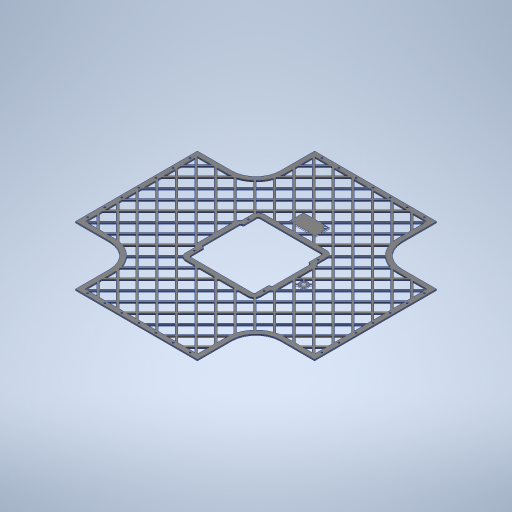
# Autodesk Inventor part: Swerve-Electronic-Pannel
Saved by Autodesk Inventor 2024.2 (Build 282272000, 272)
## iProperties
Created: 2024-01-04
Part Number: Swerve-Electronic-Pannel
Material: Aluminum 6061
Document SubType Name: Modeling
Designer: rohan
Density: 2.7 g/cm^3
Appearance: Aluminum - Flat
Author: rohan
Autodesk Inventor part; units mm, degrees
(part 1 of 6)
ref_plane "YZ Plane" through (0, 0, 0) normal (1, 0, 0) x (0, 1, 0)
ref_plane "XZ Plane" through (0, 0, 0) normal (0, 1, 0) x (-1, 0, 0)
ref_plane "XY Plane" through (0, 0, 0) normal (0, 0, 1) x (1, 0, 0)
sketch "Sketch6" plane through (0, 0, 0) normal (0, 1, 0) x (-1, 0, 0)
  line L0 (311.15, 311.15) -> (-311.15, 311.15)
  line L1 (-311.15, 311.15) -> (-311.15, -311.15)
  line L2 (-311.15, -311.15) -> (311.15, -311.15)
  line L3 (311.15, -311.15) -> (311.15, 311.15)
  line L4 (311.15, 311.15) -> (-311.15, -311.15) construction
  line L5 (-311.15, 311.15) -> (311.15, -311.15) construction
  point P0 (0, 0)
  dimension "d60" = 622.3
  dimension "d61" = 622.3
  constraints: 12 end point, 2 midpoint, 2 parallel, 1 horizontal, 1 perpendicular
  measures "d60" distance of L2.end L1.end
  measures "d61" distance of L1.end L0.end
extrude "Extrusion5" add sketch "Sketch6" along normal blind 3.175
sketch "Sketch7" plane through (0, 3.175, 0) normal (0, 1, 0) x (1, 0, 0)
  line L0 (311.15, -311.15) -> (311.15, 311.15) projected
  line L1 (311.15, 311.15) -> (-311.15, 311.15) projected
  line L2 (-311.15, 311.15) -> (-311.15, -311.15) projected
  line L3 (-311.15, -311.15) -> (311.15, -311.15) projected
  line L4 (-298.45, -298.45) -> (-298.45, 298.45)
  line L5 (-298.45, 298.45) -> (298.45, 298.45)
  line L6 (298.45, 298.45) -> (298.45, -298.45)
  line L7 (298.45, -298.45) -> (-298.45, -298.45)
  line L8 (0, -298.45) -> (0, -311.15)
  circle A0 centre (0, -304.8) radius 1.9939
  circle A1 centre (44.45, -304.8) radius 1.9939
  circle A2 centre (88.9, -304.8) radius 1.9939
  circle A3 centre (133.35, -304.8) radius 1.9939
  circle A4 centre (-44.45, -304.8) radius 1.9939
  circle A5 centre (0, -304.8) radius 1.9939
  circle A6 centre (44.45, -304.8) radius 1.9939
  circle A7 centre (88.9, -304.8) radius 1.9939
  circle A8 centre (-88.9, -304.8) radius 1.9939
  circle A9 centre (-44.45, -304.8) radius 1.9939
  circle A10 centre (0, -304.8) radius 1.9939
  circle A11 centre (44.45, -304.8) radius 1.9939
  circle A12 centre (-133.35, -304.8) radius 1.9939
  circle A13 centre (-88.9, -304.8) radius 1.9939
  circle A14 centre (-44.45, -304.8) radius 1.9939
  circle A15 centre (0, -304.8) radius 1.9939
  line L9 (-413.2249, 0) -> (395.3055, 0)
  line L10 (298.45, 298.45) -> (-298.45, 298.45)
  line L11 (0, 298.45) -> (0, 311.15)
  circle A16 centre (0, 304.8) radius 1.9939
  circle A17 centre (44.45, 304.8) radius 1.9939
  circle A18 centre (88.9, 304.8) radius 1.9939
  circle A19 centre (133.35, 304.8) radius 1.9939
  circle A20 centre (-44.45, 304.8) radius 1.9939
  circle A21 centre (0, 304.8) radius 1.9939
  circle A22 centre (44.45, 304.8) radius 1.9939
  circle A23 centre (88.9, 304.8) radius 1.9939
  circle A24 centre (-88.9, 304.8) radius 1.9939
  circle A25 centre (-44.45, 304.8) radius 1.9939
  circle A26 centre (0, 304.8) radius 1.9939
  circle A27 centre (44.45, 304.8) radius 1.9939
  circle A28 centre (-133.35, 304.8) radius 1.9939
  circle A29 centre (-88.9, 304.8) radius 1.9939
  circle A30 centre (-44.45, 304.8) radius 1.9939
  circle A31 centre (0, 304.8) radius 1.9939
  line L12 (-311.15, 0) -> (-298.45, 0)
  circle A32 centre (-304.8, 0) radius 1.9939
  circle A33 centre (-304.8, -44.45) radius 1.9939
  circle A34 centre (-304.8, -88.9) radius 1.9939
  circle A35 centre (-304.8, -133.35) radius 1.9939
  circle A36 centre (-304.8, 44.45) radius 1.9939
  circle A37 centre (-304.8, 0) radius 1.9939
  circle A38 centre (-304.8, -44.45) radius 1.9939
  circle A39 centre (-304.8, -88.9) radius 1.9939
  circle A40 centre (-304.8, 88.9) radius 1.9939
  circle A41 centre (-304.8, 44.45) radius 1.9939
  circle A42 centre (-304.8, 0) radius 1.9939
  circle A43 centre (-304.8, -44.45) radius 1.9939
  circle A44 centre (-304.8, 133.35) radius 1.9939
  circle A45 centre (-304.8, 88.9) radius 1.9939
  circle A46 centre (-304.8, 44.45) radius 1.9939
  circle A47 centre (-304.8, 0) radius 1.9939
  line L13 (0, 372.2506) -> (0, -355.6631)
  circle A48 centre (304.8, 0) radius 1.9939
  circle A49 centre (304.8, -44.45) radius 1.9939
  circle A50 centre (304.8, -88.9) radius 1.9939
  circle A51 centre (304.8, -133.35) radius 1.9939
  circle A52 centre (304.8, 44.45) radius 1.9939
  circle A53 centre (304.8, 0) radius 1.9939
  circle A54 centre (304.8, -44.45) radius 1.9939
  circle A55 centre (304.8, -88.9) radius 1.9939
  circle A56 centre (304.8, 88.9) radius 1.9939
  circle A57 centre (304.8, 44.45) radius 1.9939
  circle A58 centre (304.8, 0) radius 1.9939
  circle A59 centre (304.8, -44.45) radius 1.9939
  circle A60 centre (304.8, 133.35) radius 1.9939
  circle A61 centre (304.8, 88.9) radius 1.9939
  circle A62 centre (304.8, 44.45) radius 1.9939
  circle A63 centre (304.8, 0) radius 1.9939
  point P0 (0, 0)
  dimension "d64" = 12.7
  dimension "d65" = 3.9878
  dimension "d68" = 44.45
  dimension "d71" = 44.45
  dimension "d74" = 3.9878
  dimension "d77" = 44.45
  dimension "d80" = 44.45
  constraints: 64 centre point, 34 symmetric about line, 20 end point, 6 midpoint, 3 horizontal, 2 point on line, 2 vertical, 1 perpendicular, 95 other
  measures "d64" distance between parallel lines of L2 L4
  measures "d65" diameter of A0
  measures "d68" distance of A0.centre A1.centre
  measures "d71" distance of A0.centre A4.centre
  measures "d74" diameter of A32
  measures "d77" distance of A32.centre A33.centre
  measures "d80" distance of A32.centre A36.centre
extrude "Extrusion6" cut sketch "Sketch7" against normal blind 3.175 contours A48 L9 | L9 A48 | A0 L8 | L8 A0 | A16 L11 | L11 A16 | A32 L9 | L9 A32 | A1 | A2 | A3 | A4 | A8 | A12 | A17 | A18 | A19 | A20 | A24 | A28 | A33 | A34 | A35 | A36 | A40 | A44 | A49 | A50 | A51 | A52 | A56 | A60
sketch "Sketch8" plane through (0, 3.175, 0) normal (0, 1, 0) x (1, 0, 0)
  line L0 (-311.15, 311.15) -> (-311.15, -311.15) projected
  circle A0 centre (-304.8, 88.9) radius 1.9939 projected
  circle A1 centre (-304.8, -133.35) radius 1.9939 projected
  circle A2 centre (0, -304.8) radius 1.9939 projected
  circle A3 centre (304.8, -133.35) radius 1.9939 projected
  circle A4 centre (304.8, 44.45) radius 1.9939 projected
  circle A5 centre (88.9, 304.8) radius 1.9939 projected
  circle A6 centre (-88.9, 304.8) radius 1.9939 projected
  circle A7 centre (-44.45, 304.8) radius 1.9939 projected
  circle A8 centre (133.35, 304.8) radius 1.9939 projected
  circle A9 centre (304.8, 0) radius 1.9939 projected
  circle A10 centre (133.35, -304.8) radius 1.9939 projected
  circle A11 centre (-44.45, -304.8) radius 1.9939 projected
  circle A12 centre (-304.8, -88.9) radius 1.9939 projected
  circle A13 centre (-304.8, 133.35) radius 1.9939 projected
  circle A14 centre (-304.8, 44.45) radius 1.9939 projected
  circle A15 centre (-133.35, -304.8) radius 1.9939 projected
  circle A16 centre (44.45, -304.8) radius 1.9939 projected
  circle A17 centre (304.8, -88.9) radius 1.9939 projected
  circle A18 centre (304.8, 88.9) radius 1.9939 projected
  circle A19 centre (44.45, 304.8) radius 1.9939 projected
  circle A20 centre (-133.35, 304.8) radius 1.9939 projected
  circle A21 centre (0, 304.8) radius 1.9939 projected
  circle A22 centre (304.8, 133.35) radius 1.9939 projected
  circle A23 centre (304.8, -44.45) radius 1.9939 projected
  circle A24 centre (88.9, -304.8) radius 1.9939 projected
  circle A25 centre (-88.9, -304.8) radius 1.9939 projected
  circle A26 centre (-304.8, -44.45) radius 1.9939 projected
  circle A27 centre (-304.8, 0) radius 1.9939 projected
  line L1 (311.15, -311.15) -> (311.15, 311.15) projected
  line L2 (311.15, 311.15) -> (-311.15, 311.15) projected
  line L3 (-311.15, 311.15) -> (-311.15, -311.15) projected
  line L4 (-311.15, -311.15) -> (311.15, -311.15) projected
  line L5 (311.15, 311.15) -> (-311.15, 311.15) projected
  line L6 (-158.75, 311.15) -> (-158.75, 222.25)
  line L7 (-222.25, 158.75) -> (-311.15, 158.75)
  line L8 (-311.15, -158.75) -> (-222.25, -158.75)
  line L9 (-158.75, -222.25) -> (-158.75, -311.15)
  line L10 (158.75, 311.15) -> (158.75, 222.25)
  line L11 (222.25, 158.75) -> (311.15, 158.75)
  line L12 (158.75, -311.15) -> (158.75, -222.25)
  line L13 (222.25, -158.75) -> (311.15, -158.75)
  arc A28 (-222.25, 158.75) -> (-158.75, 222.25) centre (-222.25, 222.25) ccw
  arc A29 (158.75, 222.25) -> (222.25, 158.75) centre (222.25, 222.25) ccw
  arc A30 (222.25, -158.75) -> (158.75, -222.25) centre (222.25, -222.25) ccw
  arc A31 (-158.75, -222.25) -> (-222.25, -158.75) centre (-222.25, -222.25) ccw
  point P0 (0, 0)
  point P1 (-311.15, 0)
  point P2 (0, 311.15)
  point P3 (-158.75, 158.75)
  point P4 (-158.75, -158.75)
  point P5 (158.75, 158.75)
  point P6 (0, -311.15)
  point P7 (158.75, -158.75)
  dimension "d93" = 63.5
  constraints: 18 point on line, 16 end point, 8 point on circle, 8 tangent, 4 centre point, 3 equal radius, 3 midpoint, 2 parallel, 2 perpendicular, 2 vertical
  measures "d93" radius of A28
extrude "Extrusion8" cut sketch "Sketch8" against normal blind 61.9125 contours L2 L6 A28 L7 L0 | L8 A31 L9 L4 L0 | L2 L1 L11 A29 L10 | L12 A30 L13 L1 L4
sketch "Sketch9" plane through (0, 3.175, 0) normal (0, 1, 0) x (1, 0, 0)
  circle A0 centre (-304.8, 0) radius 1.9939 projected
  circle A1 centre (-304.8, -44.45) radius 1.9939 projected
  circle A2 centre (-88.9, -304.8) radius 1.9939 projected
  circle A3 centre (88.9, -304.8) radius 1.9939 projected
  circle A4 centre (304.8, -44.45) radius 1.9939 projected
  circle A5 centre (304.8, 133.35) radius 1.9939 projected
  circle A6 centre (0, 304.8) radius 1.9939 projected
  circle A7 centre (-133.35, 304.8) radius 1.9939 projected
  circle A8 centre (44.45, 304.8) radius 1.9939 projected
  circle A9 centre (304.8, 88.9) radius 1.9939 projected
  circle A10 centre (304.8, -88.9) radius 1.9939 projected
  circle A11 centre (44.45, -304.8) radius 1.9939 projected
  circle A12 centre (-133.35, -304.8) radius 1.9939 projected
  circle A13 centre (-304.8, 44.45) radius 1.9939 projected
  circle A14 centre (-304.8, 133.35) radius 1.9939 projected
  circle A15 centre (-304.8, -88.9) radius 1.9939 projected
  circle A16 centre (-44.45, -304.8) radius 1.9939 projected
  circle A17 centre (133.35, -304.8) radius 1.9939 projected
  circle A18 centre (304.8, 0) radius 1.9939 projected
  circle A19 centre (133.35, 304.8) radius 1.9939 projected
  circle A20 centre (-44.45, 304.8) radius 1.9939 projected
  circle A21 centre (-88.9, 304.8) radius 1.9939 projected
  circle A22 centre (88.9, 304.8) radius 1.9939 projected
  circle A23 centre (304.8, 44.45) radius 1.9939 projected
  circle A24 centre (304.8, -133.35) radius 1.9939 projected
  circle A25 centre (0, -304.8) radius 1.9939 projected
  circle A26 centre (-304.8, -133.35) radius 1.9939 projected
  circle A27 centre (-304.8, 88.9) radius 1.9939 projected
  line L0 (-311.15, -158.75) -> (-222.25, -158.75) projected
  arc A28 (-158.75, -222.25) -> (-222.25, -158.75) centre (-222.25, -222.25) ccw projected
  line L1 (-158.75, -222.25) -> (-158.75, -311.15) projected
  line L2 (-158.75, -311.15) -> (158.75, -311.15) projected
  line L3 (158.75, -311.15) -> (158.75, -222.25) projected
  arc A29 (222.25, -158.75) -> (158.75, -222.25) centre (222.25, -222.25) ccw projected
  line L4 (222.25, -158.75) -> (311.15, -158.75) projected
  line L5 (311.15, -158.75) -> (311.15, 158.75) projected
  line L6 (311.15, 158.75) -> (222.25, 158.75) projected
  arc A30 (158.75, 222.25) -> (222.25, 158.75) centre (222.25, 222.25) ccw projected
  line L7 (158.75, 222.25) -> (158.75, 311.15) projected
  line L8 (158.75, 311.15) -> (-158.75, 311.15) projected
  line L9 (-158.75, 311.15) -> (-158.75, 222.25) projected
  arc A31 (-222.25, 158.75) -> (-158.75, 222.25) centre (-222.25, 222.25) ccw projected
  line L10 (-222.25, 158.75) -> (-311.15, 158.75) projected
  line L11 (-311.15, 158.75) -> (-311.15, -158.75) projected
  line L12 (298.45, -146.05) -> (222.25, -146.05)
  arc A32 (222.25, -146.05) -> (146.05, -222.25) centre (222.25, -222.25) ccw
  line L13 (146.05, -222.25) -> (146.05, -298.45)
  line L14 (146.05, -298.45) -> (-146.05, -298.45)
  line L15 (-146.05, -298.45) -> (-146.05, -222.25)
  arc A33 (-146.05, -222.25) -> (-222.25, -146.05) centre (-222.25, -222.25) ccw
  line L16 (-222.25, -146.05) -> (-298.45, -146.05)
  line L17 (-298.45, -146.05) -> (-298.45, 146.05)
  line L18 (-298.45, 146.05) -> (-222.25, 146.05)
  arc A34 (-222.25, 146.05) -> (-146.05, 222.25) centre (-222.25, 222.25) ccw
  line L19 (-146.05, 222.25) -> (-146.05, 298.45)
  line L20 (-146.05, 298.45) -> (146.05, 298.45)
  line L21 (146.05, 298.45) -> (146.05, 222.25)
  arc A35 (146.05, 222.25) -> (222.25, 146.05) centre (222.25, 222.25) ccw
  line L22 (222.25, 146.05) -> (298.45, 146.05)
  line L23 (298.45, 146.05) -> (298.45, -146.05)
  line L24 (-129.2013, 279.4426) -> (-110.1939, 298.45)
  line L25 (-129.2013, 279.4426) -> (-102.3208, 279.4426) construction
  line L26 (-129.2013, 279.4426) -> (-146.05, 262.5939)
  line L27 (-142.4579, 259.0018) -> (-125.6092, 275.8505)
  line L28 (-125.6092, 275.8505) -> (-106.6018, 294.8579)
  line L29 (-110.1939, 291.2658) -> (-103.0097, 298.45)
  line L30 (-138.8658, 262.5939) -> (-146.05, 255.4097)
  line L31 (-146.05, 298.45) -> (-138.8658, 291.2658)
  line L32 (-103.6974, 253.9386) -> (-84.69, 272.9461)
  line L33 (-103.6974, 253.9386) -> (-120.5461, 237.09)
  line L34 (-113.3619, 237.09) -> (-120.5461, 229.9058)
  line L35 (-116.954, 233.4979) -> (-100.1053, 250.3465)
  line L36 (-100.1053, 250.3465) -> (-81.0979, 269.354)
  line L37 (-84.69, 265.7619) -> (-77.5058, 272.9461)
  line L38 (-78.1935, 228.4347) -> (-59.186, 247.4421)
  line L39 (-78.1935, 228.4347) -> (-95.0421, 211.586)
  line L40 (-87.8579, 211.586) -> (-95.0421, 204.4018)
  line L41 (-91.45, 207.9939) -> (-74.6014, 224.8426)
  line L42 (-74.6014, 224.8426) -> (-55.5939, 243.85)
  line L43 (-59.186, 240.2579) -> (-52.0018, 247.4421)
  line L44 (-52.6895, 202.9308) -> (-33.6821, 221.9382)
  line L45 (-52.6895, 202.9308) -> (-69.5382, 186.0821)
  line L46 (-62.354, 186.0821) -> (-69.5382, 178.8979)
  line L47 (-65.9461, 182.49) -> (-49.0974, 199.3387)
  line L48 (-49.0974, 199.3387) -> (-30.09, 218.3461)
  line L49 (-33.6821, 214.754) -> (-26.4979, 221.9382)
  line L50 (-27.1856, 177.4269) -> (-8.1782, 196.4343)
  line L51 (-27.1856, 177.4269) -> (-44.0343, 160.5782)
  line L52 (-36.8501, 160.5782) -> (-44.0343, 153.394)
  line L53 (-40.4422, 156.9861) -> (-23.5935, 173.8348)
  line L54 (-23.5935, 173.8348) -> (-4.5861, 192.8422)
  line L55 (-8.1782, 189.2501) -> (-0.994, 196.4343)
  line L56 (-1.6817, 151.9229) -> (17.3257, 170.9304)
  line L57 (-1.6817, 151.9229) -> (-18.5304, 135.0743)
  line L58 (-11.3462, 135.0743) -> (-18.5304, 127.8901)
  line L59 (-14.9383, 131.4822) -> (1.9104, 148.3308)
  line L60 (1.9104, 148.3308) -> (20.9178, 167.3383)
  line L61 (17.3257, 163.7462) -> (24.5099, 170.9304)
  line L62 (23.8222, 126.419) -> (42.8297, 145.4264)
  line L63 (23.8222, 126.419) -> (6.9736, 109.5703)
  line L64 (14.1578, 109.5703) -> (6.9736, 102.3861)
  line L65 (10.5657, 105.9782) -> (27.4143, 122.8269)
  line L66 (27.4143, 122.8269) -> (46.4218, 141.8343)
  line L67 (42.8297, 138.2422) -> (50.0139, 145.4264)
  line L68 (49.3262, 100.9151) -> (68.3336, 119.9225)
  line L69 (49.3262, 100.9151) -> (32.4775, 84.0664)
  line L70 (39.6617, 84.0664) -> (32.4775, 76.8822)
  line L71 (36.0696, 80.4743) -> (52.9183, 97.323)
  line L72 (52.9183, 97.323) -> (71.9257, 116.3304)
  line L73 (68.3336, 112.7383) -> (75.5178, 119.9225)
  line L74 (74.8301, 75.4112) -> (93.8375, 94.4186)
  line L75 (74.8301, 75.4112) -> (57.9814, 58.5625)
  line L76 (65.1656, 58.5625) -> (57.9814, 51.3783)
  line L77 (61.5735, 54.9704) -> (78.4222, 71.8191)
  line L78 (78.4222, 71.8191) -> (97.4296, 90.8265)
  line L79 (93.8375, 87.2344) -> (101.0217, 94.4186)
  line L80 (100.334, 49.9072) -> (119.3414, 68.9147)
  line L81 (100.334, 49.9072) -> (83.4853, 33.0586)
  line L82 (90.6696, 33.0586) -> (83.4853, 25.8743)
  line L83 (87.0774, 29.4665) -> (103.9261, 46.3151)
  line L84 (103.9261, 46.3151) -> (122.9335, 65.3226)
  line L85 (119.3414, 61.7304) -> (126.5257, 68.9147)
  line L86 (125.8379, 24.4033) -> (144.8454, 43.4107)
  line L87 (125.8379, 24.4033) -> (108.9893, 7.5546)
  line L88 (116.1735, 7.5546) -> (108.9893, 0.3704)
  line L89 (112.5814, 3.9625) -> (129.4301, 20.8112)
  line L90 (129.4301, 20.8112) -> (148.4375, 39.8186)
  line L91 (144.8454, 36.2265) -> (152.0296, 43.4107)
  line L92 (151.3419, -1.1006) -> (170.3493, 17.9068)
  line L93 (151.3419, -1.1006) -> (134.4932, -17.9493)
  line L94 (141.6774, -17.9493) -> (134.4932, -25.1335)
  line L95 (138.0853, -21.5414) -> (154.934, -4.6927)
  line L96 (154.934, -4.6927) -> (173.9414, 14.3147)
  line L97 (170.3493, 10.7226) -> (177.5335, 17.9068)
  line L98 (176.8458, -26.6046) -> (195.8532, -7.5971)
  line L99 (176.8458, -26.6046) -> (159.9971, -43.4532)
  line L100 (167.1813, -43.4532) -> (159.9971, -50.6374)
  line L101 (163.5892, -47.0453) -> (180.4379, -30.1967)
  line L102 (180.4379, -30.1967) -> (199.4453, -11.1892)
  line L103 (195.8532, -14.7813) -> (203.0374, -7.5971)
  line L104 (202.3497, -52.1085) -> (221.3572, -33.1011)
  line L105 (202.3497, -52.1085) -> (185.5011, -68.9572)
  line L106 (192.6853, -68.9572) -> (185.5011, -76.1414)
  line L107 (189.0932, -72.5493) -> (205.9418, -55.7006)
  line L108 (205.9418, -55.7006) -> (224.9493, -36.6932)
  line L109 (221.3572, -40.2853) -> (228.5414, -33.1011)
  line L110 (227.8537, -77.6124) -> (246.8611, -58.605)
  line L111 (227.8537, -77.6124) -> (211.005, -94.4611)
  line L112 (218.1892, -94.4611) -> (211.005, -101.6453)
  line L113 (214.5971, -98.0532) -> (231.4458, -81.2045)
  line L114 (231.4458, -81.2045) -> (250.4532, -62.1971)
  line L115 (246.8611, -65.7892) -> (254.0453, -58.605)
  line L116 (253.3576, -103.1163) -> (272.365, -84.1089)
  line L117 (253.3576, -103.1163) -> (236.5089, -119.965)
  line L118 (243.6931, -119.965) -> (236.5089, -127.1492)
  line L119 (240.101, -123.5571) -> (256.9497, -106.7084)
  line L120 (256.9497, -106.7084) -> (275.9571, -87.701)
  line L121 (272.365, -91.2931) -> (279.5492, -84.1089)
  line L122 (278.8615, -128.6203) -> (297.8689, -109.6128)
  line L123 (278.8615, -128.6203) -> (262.0128, -145.4689)
  line L124 (269.197, -145.4689) -> (262.0128, -152.6531)
  line L125 (265.6049, -149.061) -> (282.4536, -132.2124)
  line L126 (282.4536, -132.2124) -> (301.461, -113.2049)
  line L127 (297.8689, -116.797) -> (305.0531, -109.6128)
  line L128 (304.3654, -154.1242) -> (323.3729, -135.1168)
  line L129 (304.3654, -154.1242) -> (287.5168, -170.9729)
  line L130 (294.701, -170.9729) -> (287.5168, -178.1571)
  line L131 (291.1089, -174.565) -> (307.9575, -157.7163)
  line L132 (307.9575, -157.7163) -> (326.965, -138.7089)
  line L133 (323.3729, -142.301) -> (330.5571, -135.1168)
  line L134 (329.8694, -179.6281) -> (348.8768, -160.6207)
  line L135 (329.8694, -179.6281) -> (313.0207, -196.4768)
  line L136 (320.2049, -196.4768) -> (313.0207, -203.661)
  line L137 (316.6128, -200.0689) -> (333.4615, -183.2202)
  line L138 (333.4615, -183.2202) -> (352.4689, -164.2128)
  line L139 (348.8768, -167.8049) -> (356.061, -160.6207)
  line L140 (-84.69, 272.9461) -> (-59.186, 298.45)
  line L141 (-59.186, 298.45) -> (-146.9294, 210.7066)
  line L142 (-120.5461, 229.9058) -> (-52.0018, 298.45)
  line L143 (-52.0018, 298.45) -> (-148.9209, 201.531)
  line L144 (-95.0421, 211.586) -> (-8.1782, 298.45)
  line L145 (-8.1782, 298.45) -> (-298.45, 8.1782)
  line L146 (-52.0018, 247.4421) -> (-0.994, 298.45)
  line L147 (-0.994, 298.45) -> (-298.45, 0.994)
  line L148 (-69.5382, 186.0821) -> (-298.45, -42.8297)
  line L149 (-298.45, -42.8297) -> (42.8297, 298.45)
  line L150 (-26.4979, 221.9382) -> (50.0139, 298.45)
  line L151 (50.0139, 298.45) -> (-298.45, -50.0139)
  line L152 (-8.1782, 196.4343) -> (93.8375, 298.45)
  line L153 (93.8375, 298.45) -> (-298.45, -93.8375)
  line L154 (-44.0343, 153.394) -> (-298.45, -101.0217)
  line L155 (-298.45, -101.0217) -> (101.0217, 298.45)
  line L156 (17.3257, 170.9304) -> (144.8454, 298.45)
  line L157 (144.8454, 298.45) -> (-298.45, -144.8454)
  line L158 (-18.5304, 127.8901) -> (-292.4704, -146.05)
  line L159 (24.5099, 170.9304) -> (146.05, 292.4704)
  line L160 (42.8297, 145.4264) -> (146.05, 248.6468)
  line L161 (6.9736, 109.5703) -> (-248.6468, -146.05)
  line L162 (6.9736, 102.3861) -> (-241.4626, -146.05)
  line L163 (50.0139, 145.4264) -> (146.05, 241.4626)
  line L164 (68.3336, 119.9225) -> (149.1495, 200.7384)
  line L165 (75.5178, 119.9225) -> (150.9531, 195.3578)
  line L166 (93.8375, 94.4186) -> (168.0787, 168.6598)
  line L167 (101.0217, 94.4186) -> (171.7713, 165.1681)
  line L168 (101.0217, 94.4186) -> (201.0767, 94.4186) construction
  line L169 (171.7713, 165.1681) -> (-165.1681, -171.7713)
  line L170 (57.9814, 58.5625) -> (-168.6598, -168.0787)
  line L171 (32.4775, 84.0664) -> (-200.7384, -149.1495)
  line L172 (32.4775, 84.0664) -> (362.2945, 84.0664) construction
  line L173 (36.0696, 80.4743) -> (-195.3578, -150.9531)
  line L174 (36.0696, 80.4743) -> (363.3574, 80.4743) construction
  line L175 (122.9335, 65.3226) -> (205.5202, 147.9092)
  line L176 (205.5202, 147.9092) -> (-147.9092, -205.5202)
  line L177 (119.3414, 68.9147) -> (199.8451, 149.4183)
  line L178 (98.0319, 47.6051) -> (-149.4183, -199.8451)
  line L179 (138.9338, 30.3149) -> (254.6689, 146.05)
  line L180 (254.6689, 146.05) -> (-146.05, -254.6689)
  line L181 (144.8454, 43.4107) -> (247.4846, 146.05)
  line L182 (247.4846, 146.05) -> (-146.05, -247.4846)
  line L183 (144.8454, -7.5971) -> (-146.05, -298.4925)
  line L184 (134.4932, -25.1335) -> (-138.8233, -298.45)
  line L185 (170.3493, 10.7226) -> (298.45, 138.8233)
  line L186 (159.5933, 7.1508) -> (298.45, 146.05)
  line L187 (185.1011, -18.3493) -> (298.45, 94.9996)
  line L188 (199.4453, -11.1892) -> (298.45, 87.8154)
  line L189 (170.3493, -33.1011) -> (-94.9996, -298.45)
  line L190 (167.1813, -43.4532) -> (-87.8154, -298.45)
  line L191 (195.8532, -58.605) -> (-43.9918, -298.45)
  line L192 (195.8532, -65.7892) -> (-36.8076, -298.45)
  line L193 (214.5971, -39.8611) -> (298.45, 43.9918)
  line L194 (218.1892, -43.4532) -> (298.45, 36.8076)
  line L195 (237.3574, -68.1087) -> (298.45, -7.0161)
  line L196 (246.8611, -65.7892) -> (298.45, -14.2003)
  line L197 (265.6049, -90.869) -> (298.45, -58.0239)
  line L198 (272.365, -91.2931) -> (298.45, -65.2081)
  line L199 (296.8378, -110.644) -> (298.45, -109.0318)
  line L200 (262.0128, -145.4689) -> (261.4318, -146.05)
  line L201 (211.005, -94.4611) -> (7.0161, -298.45)
  line L202 (218.1892, -94.4611) -> (14.2003, -298.45)
  line L203 (262.0128, -145.4689) -> (261.4318, -146.05)
  line L204 (146.05, -261.4318) -> (109.0318, -298.45)
  line L205 (146.05, -268.616) -> (116.216, -298.45)
  line L206 (236.5089, -127.1492) -> (217.4573, -146.2009)
  line L207 (146.2009, -217.4573) -> (65.2081, -298.45)
  line L208 (236.5089, -119.965) -> (209.3187, -147.1553)
  line L209 (147.1553, -209.3187) -> (58.0239, -298.45)
  line L210 (-139.2899, 269.354) -> (-146.05, 262.5939)
  line L211 (-262.5939, 146.05) -> (-298.45, 110.1939)
  line L212 (-138.8658, 262.5939) -> (-146.05, 255.4097)
  line L213 (-255.4097, 146.05) -> (-298.45, 103.0097)
  line L214 (-135.6978, 221.9382) -> (-146.9294, 210.7066)
  line L215 (-210.7066, 146.9294) -> (-298.45, 59.186)
  line L216 (-135.6978, 214.754) -> (-148.9209, 201.531)
  line L217 (-201.531, 148.9209) -> (-298.45, 52.0018)
  line L218 (0, -331.2289) -> (0, 335.2576)
  line L219 (129.2013, 279.4426) -> (110.1939, 298.45)
  line L220 (129.2013, 279.4426) -> (102.3208, 279.4426) construction
  line L221 (129.2013, 279.4426) -> (146.05, 262.5939)
  line L222 (142.4579, 259.0018) -> (125.6092, 275.8505)
  line L223 (125.6092, 275.8505) -> (106.6018, 294.8579)
  line L224 (110.1939, 291.2658) -> (103.0097, 298.45)
  line L225 (138.8658, 262.5939) -> (146.05, 255.4097)
  line L226 (103.6974, 253.9386) -> (84.69, 272.9461)
  line L227 (103.6974, 253.9386) -> (120.5461, 237.09)
  line L228 (113.3619, 237.09) -> (120.5461, 229.9058)
  line L229 (116.954, 233.4979) -> (100.1053, 250.3465)
  line L230 (100.1053, 250.3465) -> (81.0979, 269.354)
  line L231 (84.69, 265.7619) -> (77.5058, 272.9461)
  line L232 (78.1935, 228.4347) -> (59.186, 247.4421)
  line L233 (78.1935, 228.4347) -> (95.0421, 211.586)
  line L234 (87.8579, 211.586) -> (95.0421, 204.4018)
  line L235 (91.45, 207.9939) -> (74.6014, 224.8426)
  line L236 (74.6014, 224.8426) -> (55.5939, 243.85)
  line L237 (59.186, 240.2579) -> (52.0018, 247.4421)
  line L238 (52.6895, 202.9308) -> (33.6821, 221.9382)
  line L239 (52.6895, 202.9308) -> (69.5382, 186.0821)
  line L240 (62.354, 186.0821) -> (69.5382, 178.8979)
  line L241 (65.9461, 182.49) -> (49.0974, 199.3387)
  line L242 (49.0974, 199.3387) -> (30.09, 218.3461)
  line L243 (33.6821, 214.754) -> (26.4979, 221.9382)
  line L244 (27.1856, 177.4269) -> (8.1782, 196.4343)
  line L245 (27.1856, 177.4269) -> (44.0343, 160.5782)
  line L246 (36.8501, 160.5782) -> (44.0343, 153.394)
  line L247 (40.4422, 156.9861) -> (23.5935, 173.8348)
  line L248 (23.5935, 173.8348) -> (4.5861, 192.8422)
  line L249 (8.1782, 189.2501) -> (0.994, 196.4343)
  line L250 (1.6817, 151.9229) -> (-17.3257, 170.9304)
  line L251 (1.6817, 151.9229) -> (18.5304, 135.0743)
  line L252 (11.3462, 135.0743) -> (18.5304, 127.8901)
  line L253 (14.9383, 131.4822) -> (-1.9104, 148.3308)
  line L254 (-1.9104, 148.3308) -> (-20.9178, 167.3383)
  line L255 (-17.3257, 163.7462) -> (-24.5099, 170.9304)
  line L256 (-23.8222, 126.419) -> (-42.8297, 145.4264)
  line L257 (-23.8222, 126.419) -> (-6.9736, 109.5703)
  line L258 (-14.1578, 109.5703) -> (-6.9736, 102.3861)
  line L259 (-10.5657, 105.9782) -> (-27.4143, 122.8269)
  line L260 (-27.4143, 122.8269) -> (-46.4218, 141.8343)
  line L261 (-42.8297, 138.2422) -> (-50.0139, 145.4264)
  line L262 (-49.3262, 100.9151) -> (-68.3336, 119.9225)
  line L263 (-49.3262, 100.9151) -> (-32.4775, 84.0664)
  line L264 (-39.6617, 84.0664) -> (-32.4775, 76.8822)
  line L265 (-36.0696, 80.4743) -> (-52.9183, 97.323)
  line L266 (-52.9183, 97.323) -> (-71.9257, 116.3304)
  line L267 (-68.3336, 112.7383) -> (-75.5178, 119.9225)
  line L268 (-74.8301, 75.4112) -> (-93.8375, 94.4186)
  line L269 (-74.8301, 75.4112) -> (-57.9814, 58.5625)
  line L270 (-65.1656, 58.5625) -> (-57.9814, 51.3783)
  line L271 (-61.5735, 54.9704) -> (-78.4222, 71.8191)
  line L272 (-78.4222, 71.8191) -> (-97.4296, 90.8265)
  line L273 (-93.8375, 87.2344) -> (-101.0217, 94.4186)
  line L274 (-100.334, 49.9072) -> (-119.3414, 68.9147)
  line L275 (-100.334, 49.9072) -> (-83.4853, 33.0586)
  line L276 (-90.6696, 33.0586) -> (-83.4853, 25.8743)
  line L277 (-87.0774, 29.4665) -> (-103.9261, 46.3151)
  line L278 (-103.9261, 46.3151) -> (-122.9335, 65.3226)
  line L279 (-119.3414, 61.7304) -> (-126.5257, 68.9147)
  line L280 (-125.8379, 24.4033) -> (-144.8454, 43.4107)
  line L281 (-125.8379, 24.4033) -> (-108.9893, 7.5546)
  line L282 (-116.1735, 7.5546) -> (-108.9893, 0.3704)
  line L283 (-112.5814, 3.9625) -> (-129.4301, 20.8112)
  line L284 (-129.4301, 20.8112) -> (-148.4375, 39.8186)
  line L285 (-151.3419, -1.1006) -> (-170.3493, 17.9068)
  line L286 (-151.3419, -1.1006) -> (-134.4932, -17.9493)
  line L287 (-141.6774, -17.9493) -> (-134.4932, -25.1335)
  line L288 (-138.0853, -21.5414) -> (-154.934, -4.6927)
  line L289 (-154.934, -4.6927) -> (-173.9414, 14.3147)
  line L290 (-176.8458, -26.6046) -> (-195.8532, -7.5971)
  line L291 (-176.8458, -26.6046) -> (-159.9971, -43.4532)
  line L292 (-163.5892, -47.0453) -> (-180.4379, -30.1967)
  line L293 (-180.4379, -30.1967) -> (-199.4453, -11.1892)
  line L294 (-202.3497, -52.1085) -> (-221.3572, -33.1011)
  line L295 (-189.0932, -72.5493) -> (-205.9418, -55.7006)
  line L296 (-205.9418, -55.7006) -> (-224.9493, -36.6932)
  line L297 (-221.3572, -40.2853) -> (-228.5414, -33.1011)
  line L298 (-227.8537, -77.6124) -> (-246.8611, -58.605)
  line L299 (-227.8537, -77.6124) -> (-211.005, -94.4611)
  line L300 (-214.5971, -98.0532) -> (-231.4458, -81.2045)
  line L301 (-231.4458, -81.2045) -> (-250.4532, -62.1971)
  line L302 (-246.8611, -65.7892) -> (-254.0453, -58.605)
  line L303 (-253.3576, -103.1163) -> (-272.365, -84.1089)
  line L304 (-253.3576, -103.1163) -> (-236.5089, -119.965)
  line L305 (-243.6931, -119.965) -> (-236.5089, -127.1492)
  line L306 (-240.101, -123.5571) -> (-256.9497, -106.7084)
  line L307 (-256.9497, -106.7084) -> (-275.9571, -87.701)
  line L308 (-278.8615, -128.6203) -> (-297.8689, -109.6128)
  line L309 (-278.8615, -128.6203) -> (-262.0128, -145.4689)
  line L310 (-265.6049, -149.061) -> (-282.4536, -132.2124)
  line L311 (-282.4536, -132.2124) -> (-301.461, -113.2049)
  line L312 (84.69, 272.9461) -> (59.186, 298.45)
  line L313 (59.186, 298.45) -> (146.9294, 210.7066)
  line L314 (120.5461, 229.9058) -> (52.0018, 298.45)
  line L315 (52.0018, 298.45) -> (148.9209, 201.531)
  line L316 (95.0421, 211.586) -> (8.1782, 298.45)
  line L317 (8.1782, 298.45) -> (298.45, 8.1782)
  line L318 (52.0018, 247.4421) -> (0.994, 298.45)
  line L319 (0.994, 298.45) -> (298.45, 0.994)
  line L320 (69.5382, 186.0821) -> (298.45, -42.8297)
  line L321 (298.45, -42.8297) -> (-42.8297, 298.45)
  line L322 (26.4979, 221.9382) -> (-50.0139, 298.45)
  line L323 (-50.0139, 298.45) -> (298.45, -50.0139)
  line L324 (8.1782, 196.4343) -> (-93.8375, 298.45)
  line L325 (-93.8375, 298.45) -> (298.45, -93.8375)
  line L326 (44.0343, 153.394) -> (298.45, -101.0217)
  line L327 (298.45, -101.0217) -> (-101.0217, 298.45)
  line L328 (-17.3257, 170.9304) -> (-144.8454, 298.45)
  line L329 (-144.8454, 298.45) -> (298.45, -144.8454)
  line L330 (18.5304, 127.8901) -> (292.4704, -146.05)
  line L331 (-24.5099, 170.9304) -> (-146.05, 292.4704)
  line L332 (-42.8297, 145.4264) -> (-146.05, 248.6468)
  line L333 (-6.9736, 109.5703) -> (248.6468, -146.05)
  line L334 (-6.9736, 102.3861) -> (241.4626, -146.05)
  line L335 (-50.0139, 145.4264) -> (-146.05, 241.4626)
  line L336 (-68.3336, 119.9225) -> (-149.1495, 200.7384)
  line L337 (-75.5178, 119.9225) -> (-150.9531, 195.3578)
  line L338 (-93.8375, 94.4186) -> (-168.0787, 168.6598)
  line L339 (-101.0217, 94.4186) -> (-171.7713, 165.1681)
  line L340 (-101.0217, 94.4186) -> (-201.0767, 94.4186) construction
  line L341 (-171.7713, 165.1681) -> (165.1681, -171.7713)
  line L342 (-57.9814, 58.5625) -> (168.6598, -168.0787)
  line L343 (-32.4775, 84.0664) -> (200.7384, -149.1495)
  line L344 (-32.4775, 84.0664) -> (-362.2945, 84.0664) construction
  line L345 (-36.0696, 80.4743) -> (195.3578, -150.9531)
  line L346 (-36.0696, 80.4743) -> (-363.3574, 80.4743) construction
  line L347 (-122.9335, 65.3226) -> (-205.5202, 147.9092)
  line L348 (-205.5202, 147.9092) -> (147.9092, -205.5202)
  line L349 (-119.3414, 68.9147) -> (-199.8451, 149.4183)
  line L350 (-98.0319, 47.6051) -> (149.4183, -199.8451)
  line L351 (-138.9338, 30.3149) -> (-254.6689, 146.05)
  line L352 (-254.6689, 146.05) -> (146.05, -254.6689)
  line L353 (-247.4846, 146.05) -> (146.05, -247.4846)
  line L354 (-144.8454, -7.5971) -> (146.05, -298.4925)
  line L355 (-134.4932, -25.1335) -> (138.8233, -298.45)
  line L356 (-170.3493, 10.7226) -> (-298.45, 138.8233)
  line L357 (-159.5933, 7.1508) -> (-298.45, 146.05)
  line L358 (-185.1011, -18.3493) -> (-298.45, 94.9996)
  line L359 (-199.4453, -11.1892) -> (-298.45, 87.8154)
  line L360 (-170.3493, -33.1011) -> (94.9996, -298.45)
  line L361 (-167.1813, -43.4532) -> (87.8154, -298.45)
  line L362 (-195.8532, -58.605) -> (43.9918, -298.45)
  line L363 (-195.8532, -65.7892) -> (36.8076, -298.45)
  line L364 (-214.5971, -39.8611) -> (-298.45, 43.9918)
  line L365 (-218.1892, -43.4532) -> (-298.45, 36.8076)
  line L366 (-237.3574, -68.1087) -> (-298.45, -7.0161)
  line L367 (-246.8611, -65.7892) -> (-298.45, -14.2003)
  line L368 (-265.6049, -90.869) -> (-298.45, -58.0239)
  line L369 (-272.365, -91.2931) -> (-298.45, -65.2081)
  line L370 (-211.005, -94.4611) -> (-7.0161, -298.45)
  line L371 (-218.1892, -94.4611) -> (-14.2003, -298.45)
  line L372 (-146.05, -261.4318) -> (-109.0318, -298.45)
  line L373 (-146.05, -268.616) -> (-116.216, -298.45)
  line L374 (-236.5089, -127.1492) -> (-217.4573, -146.2009)
  line L375 (-146.2009, -217.4573) -> (-65.2081, -298.45)
  line L376 (-236.5089, -119.965) -> (-209.3187, -147.1553)
  line L377 (-147.1553, -209.3187) -> (-58.0239, -298.45)
  line L378 (262.5939, 146.05) -> (298.45, 110.1939)
  line L379 (255.4097, 146.05) -> (298.45, 103.0097)
  line L380 (210.7066, 146.9294) -> (298.45, 59.186)
  line L381 (201.531, 148.9209) -> (298.45, 52.0018)
  line L382 (-195.8532, -58.605) -> (-202.3497, -52.1085)
  line L383 (-262.0128, -145.4689) -> (-261.4318, -146.05)
  line L384 (-297.8689, -109.6128) -> (-298.45, -109.0318)
  point P0 (0, 0)
  point P1 (-280.5432, -83.1149)
  point P2 (-298.45, -116.216)
  point P3 (-284.1353, -130.5307)
  point P4 (-258.6314, -105.0267)
  point P5 (-284.1353, -79.5228)
  point P6 (-280.5432, -75.9307)
  point P7 (-258.6314, -54.0189)
  point P8 (-280.5432, -32.1071)
  point P9 (-207.6235, -54.0189)
  point P10 (-229.5353, -32.1071)
  point P11 (-251.4472, -54.0189)
  point P12 (-229.5353, -75.9307)
  point P13 (-284.1353, -28.515)
  point P14 (-156.6157, -3.011)
  point P15 (-178.5275, 18.9008)
  point P16 (-200.4393, -3.011)
  point P17 (-178.5275, -24.9229)
  point P18 (-182.1196, -28.515)
  point P19 (-204.0314, -6.6031)
  point P20 (-225.9432, -28.515)
  point P21 (-204.0314, -50.4268)
  point P22 (-251.4472, -3.011)
  point P23 (-229.5353, -24.9229)
  point P24 (-207.6235, -3.011)
  point P25 (-229.5353, 18.9008)
  point P26 (-276.9511, -28.515)
  point P27 (-255.0393, -50.4268)
  point P28 (-233.1274, -28.515)
  point P29 (-255.0393, -6.6031)
  point P30 (-280.5432, -24.9229)
  point P31 (-258.6314, -3.011)
  point P32 (-280.5432, 18.9008)
  point P33 (-284.1353, 22.4929)
  point P34 (-284.1353, 73.5007)
  point P35 (-280.5432, 26.085)
  point P36 (-258.6314, 47.9968)
  point P37 (-280.5432, 69.9086)
  point P38 (-276.9511, 22.4929)
  point P39 (-255.0393, 0.5811)
  point P40 (-233.1274, 22.4929)
  point P41 (-255.0393, 44.4047)
  point P42 (-251.4472, 47.9968)
  point P43 (-229.5353, 26.085)
  point P44 (-207.6235, 47.9968)
  point P45 (-229.5353, 69.9086)
  point P46 (-225.9432, 22.4929)
  point P47 (-204.0314, 0.5811)
  point P48 (-182.1196, 22.4929)
  point P49 (-204.0314, 44.4047)
  point P50 (-200.4331, 48.0031)
  point P51 (-178.5246, 26.0879)
  point P52 (-156.6157, 47.9968)
  point P53 (-178.5275, 69.9086)
  point P54 (-225.9331, 73.5109)
  point P55 (-204.0246, 51.5957)
  point P56 (-182.1196, 73.5007)
  point P57 (-204.0314, 95.4126)
  point P58 (-251.4331, 99.0187)
  point P59 (-229.5246, 77.1035)
  point P60 (-207.6235, 99.0047)
  point P61 (-229.5353, 120.9165)
  point P62 (-276.9511, 73.5007)
  point P63 (-255.0393, 51.5889)
  point P64 (-233.1274, 73.5007)
  point P65 (-255.0393, 95.4126)
  point P66 (-280.5432, 77.0928)
  point P67 (-258.6314, 99.0047)
  point P68 (-280.5432, 120.9165)
  point P69 (-284.1353, 124.5086)
  point P70 (-280.5247, 128.1192)
  point P71 (-276.9331, 124.5266)
  point P72 (-255.0247, 102.6114)
  point P73 (-233.1274, 124.5086)
  point P74 (-229.5353, 128.1007)
  point P75 (0.994, 196.4343)
  point P76 (0, 197.4283)
  point P77 (-21.9118, 175.5165)
  point P78 (0, 153.6046)
  point P79 (21.9118, 175.5165)
  point P80 (47.4158, 201.0204)
  point P81 (25.5039, 222.9322)
  point P82 (3.5921, 201.0204)
  point P83 (25.5039, 179.1086)
  point P84 (-3.5921, 201.0204)
  point P85 (-25.5039, 222.9322)
  point P86 (-47.4158, 201.0204)
  point P87 (-25.5039, 179.1086)
  point P88 (-174.9354, -79.5228)
  point P89 (-153.0236, -101.4346)
  point P90 (-131.1117, -79.5228)
  point P91 (-153.0236, -57.611)
  point P92 (-149.4315, -105.0267)
  point P93 (-127.5196, -126.9386)
  point P94 (-105.6078, -105.0267)
  point P95 (-127.5196, -83.1149)
  point P96 (-54.6, -105.0267)
  point P97 (-76.5118, -83.1149)
  point P98 (-98.4236, -105.0267)
  point P99 (-76.5118, -126.9386)
  point P100 (-80.1039, -79.5228)
  point P101 (-102.0157, -57.611)
  point P102 (-123.9275, -79.5228)
  point P103 (-102.0157, -101.4346)
  point P104 (-105.6078, -54.0189)
  point P105 (-127.5196, -32.1071)
  point P106 (-149.4315, -54.0189)
  point P107 (-127.5196, -75.9307)
  point P108 (-174.9354, -28.515)
  point P109 (-153.0236, -50.4268)
  point P110 (-131.1117, -28.515)
  point P111 (-153.0236, -6.6031)
  point P112 (-153.0236, 0.5811)
  point P113 (-131.1117, 22.4929)
  point P114 (-153.0236, 44.4047)
  point P115 (-174.933, 22.4952)
  point P116 (-149.4315, -3.011)
  point P117 (-127.5196, -24.9229)
  point P118 (-105.6078, -3.011)
  point P119 (-127.5196, 18.9008)
  point P120 (-123.9275, -28.515)
  point P121 (-102.0157, -50.4268)
  point P122 (-80.1039, -28.515)
  point P123 (-102.0157, -6.6031)
  point P124 (-98.4236, -54.0189)
  point P125 (-76.5118, -75.9307)
  point P126 (-54.6, -54.0189)
  point P127 (-76.5118, -32.1071)
  point P128 (-54.6, -3.011)
  point P129 (-76.5118, 18.9008)
  point P130 (-98.4236, -3.011)
  point P131 (-76.5118, -24.9229)
  point P132 (-29.096, 22.4929)
  point P133 (-51.0079, 44.4047)
  point P134 (-72.9197, 22.4929)
  point P135 (-51.0079, 0.5811)
  point P136 (-29.096, -28.515)
  point P137 (-51.0079, -6.6031)
  point P138 (-72.9197, -28.515)
  point P139 (-51.0079, -50.4268)
  point P140 (-72.9197, -79.5228)
  point P141 (-51.0079, -101.4346)
  point P142 (-29.096, -79.5228)
  point P143 (-51.0079, -57.611)
  point P144 (-47.4158, -105.0267)
  point P145 (-25.5039, -126.9386)
  point P146 (-3.5921, -105.0267)
  point P147 (-25.5039, -83.1149)
  point P148 (-3.5921, -54.0189)
  point P149 (-25.5039, -32.1071)
  point P150 (-47.4158, -54.0189)
  point P151 (-25.5039, -75.9307)
  point P152 (-3.5921, -3.011)
  point P153 (-25.5039, 18.9008)
  point P154 (-47.4158, -3.011)
  point P155 (-25.5039, -24.9229)
  point P156 (47.4158, -3.011)
  point P157 (25.5039, 18.9008)
  point P158 (3.5921, -3.011)
  point P159 (25.5039, -24.9229)
  point P160 (-21.9118, 22.4929)
  point P161 (0, 0.5811)
  point P162 (21.9118, 22.4929)
  point P163 (0, 44.4047)
  point P164 (3.5921, 47.9968)
  point P165 (25.5039, 26.085)
  point P166 (47.4158, 47.9968)
  point P167 (25.5039, 69.9086)
  point P168 (-21.9118, 73.5007)
  point P169 (0, 51.5889)
  point P170 (21.9118, 73.5007)
  point P171 (0, 95.4126)
  point P172 (-3.5921, 47.9968)
  point P173 (-25.5039, 69.9086)
  point P174 (-47.4158, 47.9968)
  point P175 (-25.5039, 26.085)
  point P176 (-72.9197, 73.5007)
  point P177 (-51.0079, 51.5889)
  point P178 (-29.096, 73.5007)
  point P179 (-51.0079, 95.4126)
  point P180 (-47.4158, 99.0047)
  point P181 (-25.5039, 77.0928)
  point P182 (-3.5921, 99.0047)
  point P183 (-25.5039, 120.9165)
  point P184 (-98.4236, 47.9968)
  point P185 (-76.5118, 26.085)
  point P186 (-54.6, 47.9968)
  point P187 (-76.5118, 69.9086)
  point P188 (-102.0157, 44.4047)
  point P189 (-123.9275, 22.4929)
  point P190 (-102.0157, 0.5811)
  point P191 (-80.1039, 22.4929)
  point P192 (-102.0157, 51.5889)
  point P193 (-80.1039, 73.5007)
  point P194 (-102.0157, 95.4126)
  point P195 (-123.9275, 73.5007)
  point P196 (-127.5196, 69.9086)
  point P197 (-149.4315, 47.9968)
  point P198 (-127.5196, 26.085)
  point P199 (-105.6078, 47.9968)
  dimension "d96" = 12.7
  dimension "d97" = 25.4
  dimension "d98" = 45
  dimension "d99" = 5.08
  dimension "d102" = 36.068
  dimension "d107" = 45
  dimension "d108" = 135
  dimension "d109" = 135
  constraints: 646 end point, 246 symmetric about line, 228 point on line, 28 point on circle, 23 parallel, 6 horizontal, 4 centre point, 2 equal length, 2 midpoint, 1 perpendicular, 512 other
  measures "d96" distance between parallel lines of L4 L12
  measures "d97" distance of L19.end L24.start
  measures "d98" angle of L25 L24
  measures "d99" distance between parallel lines of L26 L27
  measures "d102" distance of L24.start L32.start
  measures "d107" angle of L168 L167
extrude "Extrusion9" cut sketch "Sketch9" against normal blind 5.08 contours L218 L321 L146 L20 | L20 L318 L149 L218 | L144 L321 L20 | L20 L149 L316 | L149 L324 L146 L322 | L218 L324 L150 | L322 L152 L218 | L150 L318 L152 L321 | L322 L144 L324 L142 L20 | L20 L314 L152 L316 L150 | L149 L44 L328 L42 L43 L146 L327 | L327 L152 L50 L328 L48 L49 L150 | L218 L250 L328 L54 L55 L155 | L327 L249 L248 L156 L56 L218 | L155 L322 L243 L242 L156 L244 L324 | L155 L318 L237 L236 L156 L238 L321 | L140 L324 L20 | L144 L38 L328 L36 L37 L142 L327 | L20 L152 L312 | L155 L314 L231 L230 L156 L232 L316 | L218 L333 L257 L158 L58 L59 | L253 L252 L330 L63 L161 L218 | L57 L157 L256 L332 L154 L52 L53 L331 L255 L254 | L60 L61 L159 L247 L246 L326 L160 L62 L329 L251 | L327 L140 L32 L328 L28 L29 L20 | L20 L224 L223 L156 L226 L312 L155 | L45 L148 L332 L147 L40 L41 L331 | L51 L153 L332 L151 L46 L47 L331 | L161 L343 L263 L158 L259 L258 L334 | L218 L343 L162 | L334 L171 L218 | L162 L64 L65 L330 L69 L171 L333 | L159 L241 L240 L323 L160 L325 L245 | L159 L235 L234 L319 L160 L320 L239 | L24 L328 L20 | L39 L145 L332 L143 L34 L35 L331 | L20 L156 L219 | L159 L229 L228 L315 L160 L317 L233 | L157 L262 L336 L154 L335 L261 L260 | L161 L342 L269 L158 L265 L264 L345 | L345 L171 L342 L162 | L218 L342 L173 | L345 L170 L218 | L173 L334 L170 L343 | L173 L70 L71 L330 L75 L170 L333 | L66 L67 L163 L326 L164 L68 L329 | L148 L336 L147 L335 | L153 L336 L151 L335 | L163 L323 L164 L325 | L163 L319 L164 L320 | L218 L363 L201 L14 | L14 L370 L192 L218 | L33 L141 L332 L19 L30 L27 L331 | L159 L222 L225 L21 L160 L313 L227 | L157 L268 L338 L154 L337 L267 L266 | L161 L350 L275 L158 L271 L270 L341 | L341 L171 L350 L162 | L341 L170 L350 L173 | L218 L350 L169 | L341 L178 L218 | L169 L345 L178 L342 | L169 L334 L178 L343 | L169 L76 L77 L330 L81 L178 L333 | L72 L73 L165 L326 L166 L74 L329 | L331 L26 L19 | L145 L336 A34 L143 L335 | L21 L221 L159 | L163 L315 A35 L164 L317 | L148 L338 L147 L337 | L153 L338 L151 L337 | L165 L323 L166 L325 | L165 L319 L166 L320 | L202 L363 L14 | L14 L192 L371 | L192 L361 L201 L362 | L218 L361 L191 | L362 L190 L218 | L191 L370 L190 L363 | L157 L274 L349 L154 L339 L273 L272 | L161 L353 L281 L158 L277 L276 L348 | L348 L171 L353 L162 | L348 L170 L353 L173 | L348 L178 L353 L169 | L218 L353 L176 | L348 L182 L218 | L176 L341 L182 L350 | L176 L345 L182 L342 | L176 L334 L182 L343 | L176 L82 L83 L330 L87 L182 L333 | L78 L79 L167 L326 L177 L80 L329 | L141 A34 L19 L335 | L145 L338 A34 L337 | L163 L21 A35 L313 | L165 A35 L166 L317 | L148 L349 L147 L339 | L153 L349 L151 L339 | L167 L323 L177 L325 | L167 L319 L177 L320 | L362 L202 L361 L209 L14 | L14 L377 L190 L371 L191 | L192 L355 L201 L360 | L360 L190 L355 L191 | L218 L355 L189 | L360 L184 L218 | L189 L362 L184 L361 | L189 L370 L184 L363 | L157 L280 L353 L154 L347 L279 L278 | L161 L354 L286 L158 L283 L282 L352 | L352 L171 L354 L162 | L352 L170 L354 L173 | L352 L178 L354 L169 | L352 L182 L354 L176 | L218 L354 L180 | L352 L183 L218 | L180 L348 L183 L353 | L180 L341 L183 L350 | L180 L345 L183 L342 | L180 L334 L183 L343 | L180 L88 L89 L330 L93 L183 L333 | L84 L85 L175 L326 L181 L86 L329 | L145 L349 A34 L339 | L167 A35 L177 L317 | L148 L353 L147 L347 | L153 L353 L151 L347 | L175 L323 L181 L325 | L175 L319 L181 L320 | L207 L361 L14 | L202 L355 L209 L360 | L14 L190 L375 | L189 L377 L184 L371 | L192 L352 L201 L354 | L354 L190 L352 L191 | L354 L184 L352 L189 | L183 L360 L180 L355 | L183 L362 L180 L361 | L183 L370 L180 L363 | L157 L285 L357 L154 L351 L284 | L161 L360 L291 L158 L288 L287 L355 | L355 L171 L360 L162 | L355 L170 L360 L173 | L355 L178 L360 L169 | L355 L182 L360 L176 | L184 L348 L189 L353 | L184 L341 L189 L350 | L184 L345 L189 L342 | L184 L334 L189 L343 | L184 L94 L95 L330 L99 L189 L333 | L90 L91 L179 L326 L186 L92 L329 | L145 L353 L217 L347 | L175 L381 L181 L317 | L148 L357 L147 L351 | L153 L357 L151 L351 | L179 L323 L186 L325 | L179 L319 L186 L320 | L360 L207 L355 L204 L14 | L202 L352 L209 L354 | L14 L372 L184 L375 L189 | L183 L377 L180 L371 | L192 L348 L201 L353 | L353 L190 L348 L191 | L182 L362 L176 L361 | L182 L370 L176 L363 | L157 L290 L358 L154 L356 L289 | L161 L362 L382 L158 L292 L361 | L361 L171 L362 L162 | L361 L170 L362 L173 | L361 L178 L362 L169 | L190 L341 L191 L350 | L190 L345 L191 L342 | L190 L334 L191 L343 | L190 L100 L101 L330 L105 L191 L333 | L96 L97 L185 L326 L187 L98 L329 | L145 L357 L217 L351 | L179 L381 L186 L317 | L148 L358 L147 L356 | L153 L358 L151 L356 | L185 L323 L187 L325 | L185 L319 L187 L320 | L205 L355 L14 | L207 L352 L13 L204 L354 | L202 L348 A32 L209 L353 | L14 L184 L373 | L183 L372 L15 L180 L375 | L182 L377 A33 L176 L371 | L192 L341 L201 L350 | L178 L370 L169 L363 | L353 L18 A34 L215 | A35 L22 L181 L380 | L157 L294 L364 L154 L359 L293 | L161 L370 L299 L158 L295 L363 | L363 L171 L370 L162 | L363 L170 L370 L173 | L192 L345 L201 L342 | L192 L334 L201 L343 | L192 L106 L107 L330 L111 L201 L333 | L102 L103 L188 L326 L193 L104 L329 | L145 L358 L217 L356 | L215 L357 L213 L18 L351 | L179 L22 L379 L186 L380 | L185 L381 L187 L317 | L148 L364 L147 L359 | L153 L364 L151 L359 | L188 L323 L193 L325 | L188 L319 L193 L320 | L354 L205 L13 L14 | L207 A32 L13 L353 | L202 L341 A32 L350 | L14 L15 L373 L183 | L182 L15 A33 L375 | L178 A33 L169 L371 | L157 L298 L366 L154 L365 L297 L296 | L161 L376 L304 L158 L300 L371 | L371 L171 A33 L376 L162 | L371 L170 A33 L173 | L202 L345 A32 L342 | L202 L334 L208 A32 L343 | L202 L112 L113 L330 L117 L208 L333 | L108 L109 L194 L326 L195 L110 L329 | L145 L364 L17 L217 L359 | L215 L358 L17 L213 L356 | L185 L379 L23 L187 L380 | L188 L381 L23 L193 L317 | L148 L366 L17 L147 L365 | L153 L366 L151 L365 | L194 L323 L195 L325 | L194 L319 L23 L195 L320 | L357 L18 L211 | L22 L186 L378 | L157 L303 L368 L154 L367 L302 L301 | L161 L16 L383 L309 L158 L306 L305 L374 | L374 A33 L16 L162 | L334 L12 A32 L206 | L206 L118 L119 L330 L123 L200 L12 L333 | L114 L115 L196 L326 L197 L116 L329 | L145 L17 L365 | L215 L17 L359 | L211 L17 L356 | L185 L23 L378 | L188 L23 L380 | L194 L23 L317 | L148 L17 L367 | L153 L368 L17 L151 L367 | L196 L323 L23 L197 L325 | L196 L23 L320 | L157 L308 L384 L17 L154 L369 L307 | L120 L121 L198 L326 L23 L199 L122 L329 | L153 L17 L369 | L16 L158 L310 | L124 L125 L330 L12 | L198 L23 L325 | L157 L17 L311 | L126 L23 L329